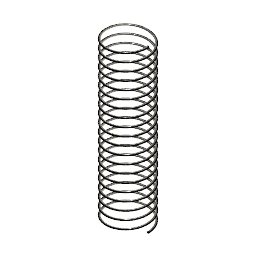
Spring (Autodesk Fusion 360 design; units mm, degrees)
Autodesk Fusion 360 part; units mm, degrees
coil "CoilPrimitive1" add diameter 5 section circle size 0.2 on centre turns 20 pitch 1 right hand placed x (1, 0, 0) y (0, 1, 0) z (0, 0, 1) at (0, 0, 0)
